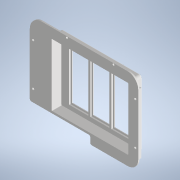
# Autodesk Inventor part: 30_XYTable_Aliexpress_sampleinsert
Saved by Autodesk Inventor 2022 (Build 260153000, 153)
## iProperties
Created: 2021-11-19
Part Number: 30_XYTable_Aliexpress_sampleinsert
Material: Generic
Document SubType Name: Modeling
Designer: diederichbenedict
Density: 1 g/cm^3
Appearance: Default
Author: diederichbenedict
Autodesk Inventor part; units mm, degrees
ref_plane "YZ Plane" through (0, 0, 0) normal (1, 0, 0) x (0, 1, 0)
ref_plane "XZ Plane" through (0, 0, 0) normal (0, 1, 0) x (-1, 0, 0)
ref_plane "XY Plane" through (0, 0, 0) normal (0, 0, 1) x (1, 0, 0)
sketch "Sketch1" plane through (0, 0, 0) normal (0, 0, 1) x (1, 0, 0)
  line L0 (53.5, -12.0505) -> (-53.5, -12.0505)
  line L1 (-57.5, -8.0505) -> (-57.5, 78.4495)
  line L2 (-53.5, 82.4495) -> (53.5, 82.4495)
  line L3 (57.5, 78.4495) -> (57.5, -8.0505)
  line L4 (57.5, -12.0505) -> (-57.5, 82.4495) construction
  line L5 (-57.5, -12.0505) -> (57.5, 82.4495) construction
  arc A0 (-53.5, 82.4495) -> (-57.5, 78.4495) centre (-53.5, 78.4495) ccw
  arc A1 (57.5, 78.4495) -> (53.5, 82.4495) centre (53.5, 78.4495) ccw
  arc A2 (53.5, -12.0505) -> (57.5, -8.0505) centre (53.5, -8.0505) ccw
  arc A3 (-57.5, -8.0505) -> (-53.5, -12.0505) centre (-53.5, -8.0505) ccw
  point P0 (0, 0)
  point P1 (0, 35.1995)
  dimension "d0" = 115
  dimension "d1" = 94.5
  dimension "d2" = 4
  constraints: 12 end point, 8 point on circle, 8 point on line, 8 tangent, 4 centre point, 3 equal radius, 2 midpoint, 2 parallel, 1 horizontal, 1 perpendicular
  measures "d0" distance of L4.end L5.end
  measures "d1" distance of L5.start L4.end
  measures "d2" radius of A0
extrude "Extrusion1" add sketch "Sketch1" along normal blind 15
sketch "Sketch2" plane through (0, 0, 15) normal (0, 0, 1) x (1, 0, 0)
  line L0 (53.5, 82.4495) -> (-53.5, 82.4495) projected
  arc A0 (-53.5, 82.4495) -> (-57.5, 78.4495) centre (-53.5, 78.4495) ccw projected
  line L1 (-57.5, 78.4495) -> (-57.5, -8.0505) projected
  arc A1 (-57.5, -8.0505) -> (-53.5, -12.0505) centre (-53.5, -8.0505) ccw projected
  line L2 (-53.5, -12.0505) -> (53.5, -12.0505) projected
  arc A2 (53.5, -12.0505) -> (57.5, -8.0505) centre (53.5, -8.0505) ccw projected
  line L3 (57.5, -8.0505) -> (57.5, 78.4495) projected
  arc A3 (57.5, 78.4495) -> (53.5, 82.4495) centre (53.5, 78.4495) ccw projected
  line L4 (-53.5, 93.4495) -> (53.5, 93.4495)
  arc A4 (68.5, 78.4495) -> (53.5, 93.4495) centre (53.5, 78.4495) ccw
  line L5 (68.5, 78.4495) -> (68.5, -8.0505)
  arc A5 (53.5, -23.0505) -> (68.5, -8.0505) centre (53.5, -8.0505) ccw
  line L6 (53.5, -23.0505) -> (-53.5, -23.0505)
  arc A6 (-68.5, -8.0505) -> (-53.5, -23.0505) centre (-53.5, -8.0505) ccw
  line L7 (-68.5, -8.0505) -> (-68.5, 78.4495)
  arc A7 (-53.5, 93.4495) -> (-68.5, 78.4495) centre (-53.5, 78.4495) ccw
  circle A8 centre (-32.5, 91.4495) radius 1.5
  circle A9 centre (33.5, 91.4495) radius 1.5
  circle A10 centre (64.5, 64.6495) radius 1.5
  circle A11 centre (64.5, 4.6495) radius 1.5
  point P0 (0, 0)
  dimension "d5" = 11
  dimension "d6" = 3
  dimension "d7" = 3
  dimension "d8" = 3
  dimension "d9" = 3
  dimension "d10" = 24
  dimension "d11" = 66
  dimension "d12" = 9
  dimension "d13" = 7
  dimension "d14" = 7
  dimension "d15" = 17.8
  dimension "d16" = 60
  constraints: 8 centre point, 8 end point, 8 point on circle, 7 other
  measures "d5" distance between parallel lines of L0 L4
  measures "d6" diameter of A8
  measures "d7" diameter of A9
  measures "d8" diameter of A10
  measures "d9" diameter of A11
  measures "d10" distance from line of A9.centre L3
  measures "d11" distance of A8.centre A9.centre
  measures "d12" distance from line of A9.centre L0
  measures "d13" distance from line of L3 A10.centre
  measures "d14" distance from line of L3 A11.centre
  measures "d15" distance from line of A10.centre L0
  measures "d16" distance of A11.centre A10.centre
extrude "Extrusion2" add sketch "Sketch2" along normal blind 2 contours A3 L3 A2 L2 A1 L1 A0 L0 | L4 A4 L5 A5 L6 A6 L7 A7
sketch "Sketch3" plane through (0, 0, 15) normal (0, 0, -1) x (-1, 0, 0)
  circle A0 centre (-64.5, 4.6495) radius 1.5 projected
  circle A1 centre (-64.5, 64.6495) radius 1.5 projected
  circle A2 centre (-33.5, 91.4495) radius 1.5 projected
  circle A3 centre (32.5, 91.4495) radius 1.5 projected
  line L0 (53.5, -23.0505) -> (-53.5, -23.0505) projected
  arc A4 (53.5, -23.0505) -> (68.5, -8.0505) centre (53.5, -8.0505) ccw projected
  line L1 (68.5, 78.4495) -> (68.5, -8.0505) projected
  arc A5 (68.5, 78.4495) -> (53.5, 93.4495) centre (53.5, 78.4495) ccw projected
  line L2 (-53.5, 93.4495) -> (53.5, 93.4495) projected
  arc A6 (-53.5, 93.4495) -> (-68.5, 78.4495) centre (-53.5, 78.4495) ccw projected
  line L3 (-68.5, -8.0505) -> (-68.5, 78.4495) projected
  arc A7 (-68.5, -8.0505) -> (-53.5, -23.0505) centre (-53.5, -8.0505) ccw projected
  arc A8 (-53.5, 82.4495) -> (-57.5, 78.4495) centre (-53.5, 78.4495) ccw projected
  line L4 (-53.5, 82.4495) -> (53.5, 82.4495) projected
  arc A9 (57.5, 78.4495) -> (53.5, 82.4495) centre (53.5, 78.4495) ccw projected
  line L5 (57.5, 78.4495) -> (57.5, -8.0505) projected
  arc A10 (53.5, -12.0505) -> (57.5, -8.0505) centre (53.5, -8.0505) ccw projected
  line L6 (53.5, -12.0505) -> (-53.5, -12.0505) projected
  arc A11 (-57.5, -8.0505) -> (-53.5, -12.0505) centre (-53.5, -8.0505) ccw projected
  line L7 (-57.5, -8.0505) -> (-57.5, 78.4495) projected
  arc A12 (-53.5, 93.4495) -> (-68.5, 78.4495) centre (-53.5, 78.4495) ccw projected
  line L8 (-57.5, -8.0505) -> (-57.5, 78.4495) projected
  line L9 (-68.5, 78.4495) -> (-57.5, 78.4495)
  line L10 (-57.5, 78.4495) -> (-57.5, -8.0505)
  line L11 (-57.5, -8.0505) -> (-68.5, -8.0505)
  line L12 (-68.5, -8.0505) -> (-68.5, 78.4495)
  point P0 (0, 0)
  point P1 (-68.5, -0.3835)
  constraints: 8 end point, 2 parallel, 1 horizontal, 1 perpendicular, 1 point on line
extrude "Extrusion3" add sketch "Sketch3" along normal blind 2.5 contours L3 L9 L7 L11
sketch "Sketch4" plane through (0, 0, 17) normal (0, 0, 1) x (1, 0, 0)
  line L0 (53.5, 82.4495) -> (-53.5, 82.4495) projected
  arc A0 (57.5, 78.4495) -> (53.5, 82.4495) centre (53.5, 78.4495) ccw projected
  line L1 (57.5, -8.0505) -> (57.5, 78.4495) projected
  arc A1 (53.5, -12.0505) -> (57.5, -8.0505) centre (53.5, -8.0505) ccw projected
  line L2 (-53.5, -12.0505) -> (53.5, -12.0505) projected
  arc A2 (-57.5, -8.0505) -> (-53.5, -12.0505) centre (-53.5, -8.0505) ccw projected
  line L3 (-57.5, 78.4495) -> (-57.5, -8.0505) projected
  arc A3 (-53.5, 82.4495) -> (-57.5, 78.4495) centre (-53.5, 78.4495) ccw projected
  line L4 (-53.5, 79.4495) -> (53.5, 79.4495)
  arc A4 (54.5, 78.4495) -> (53.5, 79.4495) centre (53.5, 78.4495) ccw
  line L5 (54.5, 78.4495) -> (54.5, -8.0505)
  arc A5 (53.5, -9.0505) -> (54.5, -8.0505) centre (53.5, -8.0505) ccw
  line L6 (53.5, -9.0505) -> (-53.5, -9.0505)
  arc A6 (-54.5, -8.0505) -> (-53.5, -9.0505) centre (-53.5, -8.0505) ccw
  line L7 (-54.5, -8.0505) -> (-54.5, 78.4495)
  arc A7 (-53.5, 79.4495) -> (-54.5, 78.4495) centre (-53.5, 78.4495) ccw
  point P0 (0, 0)
  dimension "d21" = 3
  constraints: 8 end point, 8 point on circle, 4 centre point, 7 other
  measures "d21" distance between parallel lines of L0 L4
extrude "Extrusion4" cut sketch "Sketch4" against normal blind 14 contours L4 A4 L5 A5 L6 A6 L7 A7
sketch "Sketch5" plane through (0, 0, 3) normal (0, 0, 1) x (1, 0, 0)
  line L0 (53.5, -9.0505) -> (-53.5, -9.0505) projected
  arc A0 (53.5, -9.0505) -> (54.5, -8.0505) centre (53.5, -8.0505) ccw projected
  line L1 (54.5, 78.4495) -> (54.5, -8.0505) projected
  arc A1 (54.5, 78.4495) -> (53.5, 79.4495) centre (53.5, 78.4495) ccw projected
  line L2 (-53.5, 79.4495) -> (53.5, 79.4495) projected
  arc A2 (-53.5, 79.4495) -> (-54.5, 78.4495) centre (-53.5, 78.4495) ccw projected
  line L3 (-54.5, -8.0505) -> (-54.5, 78.4495) projected
  arc A3 (-54.5, -8.0505) -> (-53.5, -9.0505) centre (-53.5, -8.0505) ccw projected
  line L4 (-53.5, 78.4495) -> (53.5, -8.0505) construction
  line L5 (53.5, -8.0505) -> (53.5, 78.4495) construction
  line L6 (53.5, -9.0505) -> (-53.5, -9.0505) construction
  arc A4 (-54.5, -8.0505) -> (-53.5, -9.0505) centre (-53.5, -8.0505) ccw construction
  line L7 (53.5, 78.4495) -> (-53.5, -8.0505) construction
  line L8 (13.5, -3.3005) -> (13.5, 73.6995)
  line L9 (13.5, 73.6995) -> (-13.5, 73.6995)
  line L10 (-13.5, 73.6995) -> (-13.5, -3.3005)
  line L11 (-13.5, -3.3005) -> (13.5, -3.3005)
  line L12 (13.5, -3.3005) -> (-13.5, 73.6995) construction
  line L13 (13.5, 73.6995) -> (-13.5, -3.3005) construction
  point P0 (0, 0)
  point P1 (0, 35.1995)
  dimension "d24" = 77
  dimension "d25" = 27
  constraints: 18 end point, 3 midpoint, 2 parallel, 2 perpendicular, 1 vertical
  measures "d24" distance between parallel lines of L11 L9
  measures "d25" distance between parallel lines of L8 L10
extrude "Extrusion5" cut sketch "Sketch5" against normal blind 2 contours L11 L10 L9 L8
sketch "Sketch6" plane through (0, 0, 1) normal (0, 0, 1) x (1, 0, 0)
  line L0 (-13.5, -3.3005) -> (-13.5, 73.6995) projected
  line L1 (-13.5, 73.6995) -> (13.5, 73.6995) projected
  line L2 (13.5, 73.6995) -> (13.5, -3.3005) projected
  line L3 (13.5, -3.3005) -> (-13.5, -3.3005) projected
  line L4 (53.5, -9.0505) -> (-53.5, -9.0505) projected
  arc A0 (53.5, -9.0505) -> (54.5, -8.0505) centre (53.5, -8.0505) ccw projected
  line L5 (54.5, 78.4495) -> (54.5, -8.0505) projected
  arc A1 (54.5, 78.4495) -> (53.5, 79.4495) centre (53.5, 78.4495) ccw projected
  line L6 (-53.5, 79.4495) -> (53.5, 79.4495) projected
  arc A2 (-53.5, 79.4495) -> (-54.5, 78.4495) centre (-53.5, 78.4495) ccw projected
  line L7 (-54.5, -8.0505) -> (-54.5, 78.4495) projected
  arc A3 (-54.5, -8.0505) -> (-53.5, -9.0505) centre (-53.5, -8.0505) ccw projected
  line L8 (-13.5, 73.6995) -> (13.5, 73.6995) projected
  line L9 (-13.5, -3.3005) -> (-13.5, 73.6995) projected
  line L10 (13.5, -3.3005) -> (-13.5, -3.3005) projected
  line L11 (13.5, 73.6995) -> (13.5, -3.3005) projected
  line L12 (-11.5, 71.6995) -> (11.5, 71.6995)
  line L13 (11.5, 71.6995) -> (11.5, -1.3005)
  line L14 (11.5, -1.3005) -> (-11.5, -1.3005)
  line L15 (-11.5, -1.3005) -> (-11.5, 71.6995)
  point P0 (0, 0)
  dimension "d28" = 2
  constraints: 8 end point, 3 other
  measures "d28" distance between parallel lines of L9 L15
extrude "Extrusion6" cut sketch "Sketch6" against normal blind 2 contours L12 L13 L14 L15
pattern_linear "Rectangular Pattern1" count 3 spacing 30 along (1, 0, 0) of "Extrusion6", "Extrusion5" first direction both ways yes
sketch "Sketch7" plane through (0, 0, 17) normal (0, 0, 1) x (1, 0, 0)
  arc A0 (53.5, -9.0505) -> (54.5, -8.0505) centre (53.5, -8.0505) ccw projected
  line L0 (53.5, -9.0505) -> (-53.5, -9.0505) projected
  arc A1 (-54.5, -8.0505) -> (-53.5, -9.0505) centre (-53.5, -8.0505) ccw projected
  line L1 (-54.5, -8.0505) -> (-54.5, 78.4495) projected
  arc A2 (-53.5, 79.4495) -> (-54.5, 78.4495) centre (-53.5, 78.4495) ccw projected
  line L2 (-53.5, 79.4495) -> (53.5, 79.4495) projected
  arc A3 (54.5, 78.4495) -> (53.5, 79.4495) centre (53.5, 78.4495) ccw projected
  line L3 (54.5, 78.4495) -> (54.5, -8.0505) projected
  line L4 (-53.5, -23.0505) -> (53.5, -23.0505) projected
  arc A4 (53.5, -23.0505) -> (68.5, -8.0505) centre (53.5, -8.0505) ccw projected
  line L5 (68.5, -8.0505) -> (68.5, 78.4495) projected
  arc A5 (68.5, 78.4495) -> (53.5, 93.4495) centre (53.5, 78.4495) ccw projected
  line L6 (53.5, 93.4495) -> (-53.5, 93.4495) projected
  arc A6 (-53.5, 93.4495) -> (-68.5, 78.4495) centre (-53.5, 78.4495) ccw projected
  line L7 (-68.5, 78.4495) -> (-68.5, -8.0505) projected
  arc A7 (-68.5, -8.0505) -> (-53.5, -23.0505) centre (-53.5, -8.0505) ccw projected
  circle A8 centre (-32.5, 91.4495) radius 1.5 projected
  circle A9 centre (33.5, 91.4495) radius 1.5 projected
  circle A10 centre (64.5, 64.6495) radius 1.5 projected
  circle A11 centre (64.5, 4.6495) radius 1.5 projected
  line L8 (-53.5, -12.0505) -> (53.5, -12.0505) projected
  line L9 (-75.3145, -26.4449) -> (0.399, -26.4449)
  line L10 (0.399, -26.4449) -> (0.399, -12.0505)
  line L11 (0.399, -12.0505) -> (-75.3145, -12.0505)
  line L12 (-75.3145, -12.0505) -> (-75.3145, -26.4449)
  point P0 (0, 0)
  constraints: 8 end point, 2 parallel, 1 horizontal, 1 perpendicular, 1 point on line
extrude "Extrusion7" cut sketch "Sketch7" against normal through all contours A7 L11 L8 L10 L4 | L4 L10 L9 L12 L11 A7
fillet "Fillet1" radius 2 11 edges at (56.3284, -10.8789, 0) (57.5, 35.1995, 0) (56.3284, 81.2779, 0) (0, 82.4495, 0) (-56.3284, 81.2779, 0) (-57.5, 35.1995, 0) (-56.3284, -10.8789, 0) (0, -12.0505, 0) (-67.9568, -12.0505, 16) (0.399, -12.0505, 16) (0.399, -23.0505, 16)
sketch "Sketch8" plane through (0, 0, 17) normal (0, 0, 1) x (1, 0, 0)
  circle A0 centre (64.5, 64.6495) radius 1.5 projected
  circle A1 centre (64.5, 4.6495) radius 1.5 projected
  circle A2 centre (-80.5, 64.6495) radius 1.5
  circle A3 centre (-80.5, 4.6495) radius 1.5
  arc A4 (0.399, -21.0505) -> (2.399, -23.0505) centre (2.399, -21.0505) ccw projected
  line L0 (2.399, -23.0505) -> (53.5, -23.0505) projected
  arc A5 (53.5, -23.0505) -> (68.5, -8.0505) centre (53.5, -8.0505) ccw projected
  line L1 (68.5, -8.0505) -> (68.5, 78.4495) projected
  arc A6 (68.5, 78.4495) -> (53.5, 93.4495) centre (53.5, 78.4495) ccw projected
  line L2 (53.5, 93.4495) -> (-53.5, 93.4495) projected
  arc A7 (-53.5, 93.4495) -> (-68.5, 78.4495) centre (-53.5, 78.4495) ccw projected
  line L3 (-68.5, 78.4495) -> (-68.5, -8.0505) projected
  arc A8 (-68.5, -8.0505) -> (-68.3214, -10.3582) centre (-53.5, -8.0505) ccw projected
  arc A9 (-68.3214, -10.3582) -> (-66.3452, -12.0505) centre (-66.3452, -10.0505) ccw projected
  line L4 (-66.3452, -12.0505) -> (-1.601, -12.0505) projected
  arc A10 (0.399, -14.0505) -> (-1.601, -12.0505) centre (-1.601, -14.0505) ccw projected
  line L5 (0.399, -14.0505) -> (0.399, -21.0505) projected
  arc A11 (53.5, -9.0505) -> (54.5, -8.0505) centre (53.5, -8.0505) ccw projected
  line L6 (53.5, -9.0505) -> (-53.5, -9.0505) projected
  arc A12 (-54.5, -8.0505) -> (-53.5, -9.0505) centre (-53.5, -8.0505) ccw projected
  line L7 (-54.5, -8.0505) -> (-54.5, 78.4495) projected
  arc A13 (-53.5, 79.4495) -> (-54.5, 78.4495) centre (-53.5, 78.4495) ccw projected
  line L8 (-53.5, 79.4495) -> (53.5, 79.4495) projected
  arc A14 (54.5, 78.4495) -> (53.5, 79.4495) centre (53.5, 78.4495) ccw projected
  line L9 (54.5, 78.4495) -> (54.5, -8.0505) projected
  circle A15 centre (-32.5, 91.4495) radius 1.5 projected
  circle A16 centre (33.5, 91.4495) radius 1.5 projected
  circle A17 centre (64.5, 64.6495) radius 1.5 projected
  circle A18 centre (64.5, 4.6495) radius 1.5 projected
  line L10 (-85.3471, -10.0505) -> (-85.3471, 76.5206)
  arc A19 (-68.4182, 93.4495) -> (-85.3471, 76.5206) centre (-68.4182, 76.5206) ccw
  line L11 (-53.5, 93.4495) -> (-68.4182, 93.4495)
  line L12 (-53.5, -12.0505) -> (-66.3452, -12.0505) projected
  line L13 (-66.3452, -12.0505) -> (-83.3471, -12.0505)
  line L14 (-85.3471, -10.0505) -> (-85.3471, -10.0505)
  arc A20 (-85.3471, -10.0505) -> (-83.3471, -12.0505) centre (-83.3471, -10.0505) ccw
  point P0 (0, 0)
  dimension "d37" = 3
  dimension "d38" = 3
  dimension "d39" = 145
  dimension "d40" = 0
  dimension "d41" = 0
  dimension "d42" = 2
  constraints: 8 end point, 4 centre point, 4 point on circle, 4 tangent, 2 horizontal, 1 perpendicular, 1 vertical
  measures "d37" diameter of A2
  measures "d38" diameter of A3
  measures "d39" distance of A2.centre A0.centre
  measures "d40" horizontal distance of A2.centre A3.centre
  measures "d41" vertical distance of A0.centre A2.centre
  measures "d42" radius of A20
extrude "Extrusion8" add sketch "Sketch8" against normal up to surface (2 mm away) contours L13 A20 L10 A19 L11 A7 L3 A8 A9
body "Solid1"
